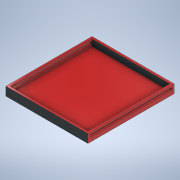
# Autodesk Inventor part: Part6
Saved by Autodesk Inventor 2020 (Build 240168000, 168)
## iProperties
Created: 2022-04-26
Part Number: Part6
Material: Iron, Cast
Document SubType Name: Modeling
Designer: Manish
Density: 7.15 g/cm^3
Appearance: Iron Gray
Mass: 238054 g
Surface Area: 28304.3 cm^2
Volume: 33294.3 cm^3
Author: Manish
Autodesk Inventor part; units mm, degrees
sketch "Sketch1" plane through (0, 0, 0) normal (0, 1, 0) x (-1, 0, 0)
  line L0 (0, 0) -> (1000, 0)
  line L1 (1000, 0) -> (1000, 1000)
  line L2 (1000, 1000) -> (0, 1000)
  line L3 (0, 1000) -> (0, 0)
  dimension "d0" = 1000
  dimension "d1" = 1000
  constraints: 8 end point, 2 parallel, 1 horizontal, 1 perpendicular
  measures "d0" distance of L2.end L1.end
  measures "d1" distance of L1.end L0.end
extrude "Extrusion1" add sketch "Sketch1" along normal blind 25.4
sketch "Sketch2" plane through (0, 0, 0) normal (1, 0, 0) x (0, 1, 0)
  line L0 (25.4, 1000) -> (25.4, 0) projected
  line L1 (25.4, 0) -> (105.4, 0)
  line L2 (105.4, 0) -> (105.4, 1000)
  line L3 (105.4, 1000) -> (25.4, 1000)
  line L4 (25.4, 1000) -> (25.4, 0)
  point P0 (0, 0)
  dimension "d4" = 80
  dimension "d5" = 1000
  constraints: 8 end point, 2 parallel, 1 horizontal, 1 perpendicular
  measures "d4" distance of L3.end L2.end
  measures "d5" distance of L2.end L1.end
extrude "Extrusion2" add sketch "Sketch2" against normal blind 25.4
sketch "Sketch3" plane through (-1000, 0, 0) normal (-1, 0, 0) x (0, 0, 1)
  line L0 (1000, 0) -> (1000, 25.4) projected
  line L1 (1000, 105.4) -> (0, 105.4) projected
  line L2 (1000, 25.4) -> (0, 25.4)
  line L3 (0, 25.4) -> (0, 105.4)
  line L4 (0, 105.4) -> (1000, 105.4)
  line L5 (1000, 105.4) -> (1000, 25.4)
  point P0 (0, 0)
  dimension "d8" = 1000
  dimension "d9" = 80
  constraints: 8 end point, 2 parallel, 1 horizontal, 1 perpendicular
  measures "d8" distance of L1.end L4.end
  measures "d9" distance of L2.end L1.end
extrude "Extrusion3" add sketch "Sketch3" against normal blind 25.4
sketch "Sketch4" plane through (-25.4, 0, 0) normal (-1, 0, 0) x (0, 0, 1)
  line L0 (0, 50.4) -> (1000, 50.4)
  line L1 (1000, 50.4) -> (1000, 80.4)
  line L2 (1000, 80.4) -> (0, 80.4)
  line L3 (0, 80.4) -> (0, 50.4)
  point P0 (0, 0)
  dimension "d12" = 1000
  dimension "d13" = 30
  constraints: 8 end point, 2 parallel, 1 horizontal, 1 perpendicular
  measures "d12" distance of L2.end L1.end
  measures "d13" distance of L1.end L0.end
extrude "Extrusion4" cut sketch "Sketch4" against normal blind 25.4
sketch "Sketch5" plane through (-974.6, 0, 0) normal (1, 0, 0) x (0, 0, -1)
  line L0 (0, 25.4) -> (0, 105.4) projected
  line L1 (0, 50.4) -> (-1000, 50.4)
  line L2 (-1000, 50.4) -> (-1000, 80.4)
  line L3 (-1000, 80.4) -> (0, 80.4)
  line L4 (0, 80.4) -> (0, 50.4)
  line L5 (0, 25.4) -> (-1000, 25.4) projected
  point P0 (0, 0)
  point P1 (0, 80.4)
  dimension "d16" = 1000
  dimension "d17" = 30
  dimension "d18" = 25
  constraints: 8 end point, 2 parallel, 1 horizontal, 1 perpendicular, 1 point on line
  measures "d16" distance of L2.end L3.end
  measures "d17" distance of L1.end L2.end
  measures "d18" distance between parallel lines of L5 L1
extrude "Extrusion5" cut sketch "Sketch5" against normal blind 25.4
ref_plane "Work Plane1" through (-1000, 65.4, 1000) normal (0, 1, 0) x (1, 0, 0)
sketch "Sketch6" plane through (-1000, 0, 1000) normal (0, 0, 1) x (1, 0, 0)
  line L0 (0, 80.4) -> (0, 105.4) projected
  line L1 (1000, 0) -> (0, 0)
  line L2 (0, 0) -> (0, 105.4)
  line L3 (0, 105.4) -> (1000, 105.4)
  line L4 (1000, 105.4) -> (1000, 0)
  constraints: 8 end point, 2 parallel, 1 horizontal, 1 perpendicular
extrude "Extrusion6" add sketch "Sketch6" along normal blind 25.4
sketch "Sketch7" plane through (0, 0, 0) normal (0, 0, -1) x (-1, 0, 0)
  line L0 (0, 105.4) -> (1000, 105.4) projected
  line L1 (0, 0) -> (1000, 0)
  line L2 (1000, 0) -> (1000, 105.4)
  line L3 (1000, 105.4) -> (0, 105.4)
  line L4 (0, 105.4) -> (0, 0)
  constraints: 8 end point, 2 parallel, 1 horizontal, 1 perpendicular
extrude "Extrusion7" add sketch "Sketch7" along normal blind 25.4
ref_plane "Work Plane2" through (-1000, 0, 500) normal (0, 0, 1) x (1, 0, 0)
ref_plane "Work Plane3" through (0, 0, 1025.4) normal (1, 0, 0) x (0, 0, -1)
body "Solid1"
